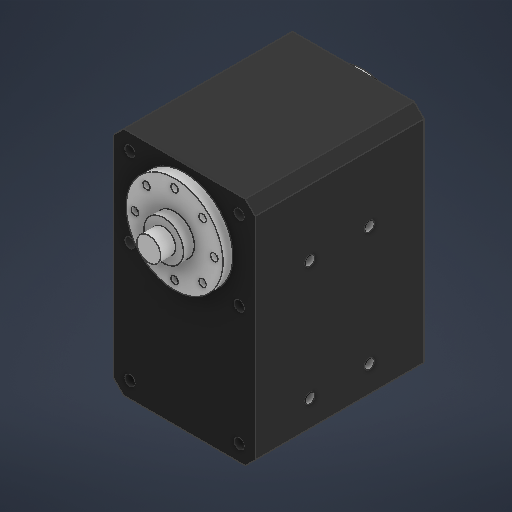
# Autodesk Inventor part: DYNAMIXEL XM430-W350
Saved by Autodesk Inventor 2025 (Build 290162010, 162A)
## iProperties
Created: 2024-06-21
Part Number: DYNAMIXEL XM430-W350
Material: Типовые
Document SubType Name: Modeling
Designer: Edward_Higgins
Density: 1 g/cm^3
Appearance: По умолчанию
Author: Edward_Higgins
Autodesk Inventor part; units mm, degrees
ref_plane "YZ Plane" through (0, 0, 0) normal (1, 0, 0) x (0, 1, 0)
ref_plane "XZ Plane" through (0, 0, 0) normal (0, 1, 0) x (-1, 0, 0)
ref_plane "XY Plane" through (0, 0, 0) normal (0, 0, 1) x (1, 0, 0)
sketch "Эскиз1" plane through (0, 0, 0) normal (0, 0, 1) x (1, 0, 0)
  line L0 (-12.25, 11.25) -> (12.25, 11.25)
  line L1 (14.25, 9.25) -> (14.25, -33.25)
  line L2 (12.25, -35.25) -> (-12.25, -35.25)
  line L3 (-14.25, -33.25) -> (-14.25, 9.25)
  circle A0 centre (-11, 8) radius 1
  circle A1 centre (-11, -8) radius 1
  circle A2 centre (11, 8) radius 1
  circle A3 centre (11, -8) radius 1
  circle A4 centre (11, -32) radius 1
  circle A5 centre (-11, -32) radius 1
  line L4 (-12.25, 11.25) -> (-14.25, 9.25)
  line L5 (12.25, 11.25) -> (14.25, 9.25)
  line L6 (14.25, -33.25) -> (12.25, -35.25)
  line L7 (-12.25, -35.25) -> (-14.25, -33.25)
  point P0 (0, 0)
  point P1 (-14.25, 11.25)
  point P2 (14.25, -35.25)
  point P3 (14.25, 11.25)
  point P4 (-14.25, -35.25)
  point P5 (0, 11.25)
  dimension "d0" = 28.5
  dimension "d1" = 46.5
  dimension "d2" = 11.25
  dimension "d3" = 22
  dimension "d4" = 11
  dimension "d5" = 8
  dimension "d6" = 8
  dimension "d7" = 40
  dimension "d8" = 2
  dimension "d11" = 2
  dimension "d12" = 2
  dimension "d13" = 2
  dimension "d14" = 2
  dimension "d15" = 2
  dimension "d16" = 2
  dimension "d17" = 2
  dimension "d18" = 2
  constraints: 16 end point, 8 point on line, 6 centre point, 5 equal radius, 5 vertical alignment, 3 horizontal alignment, 2 parallel, 1 horizontal, 1 midpoint, 1 perpendicular
  measures "d0" distance between parallel lines of L1 L3
  measures "d1" distance between parallel lines of L2 L0
  measures "d2" distance from line of point (0, 0) L0
  measures "d3" distance of A2.centre A0.centre
  measures "d4" horizontal distance of point (0, 11.25) A2.centre
  measures "d5" vertical distance of point (0, 0) A0.centre
  measures "d6" vertical distance of A1.centre point (0, 0)
  measures "d7" distance of A2.centre A4.centre
  measures "d8" diameter of A5
  measures "d11" distance of L0.start point (-14.25, 11.25)
  measures "d12" distance of L3.end point (-14.25, 11.25)
  measures "d13" distance of L0.end point (14.25, 11.25)
  measures "d14" distance of L1.start point (14.25, 11.25)
  measures "d15" distance of L1.end point (14.25, -35.25)
  measures "d16" distance of L2.start point (14.25, -35.25)
  measures "d17" distance of L2.end point (-14.25, -35.25)
  measures "d18" distance of L3.start point (-14.25, -35.25)
extrude "Выдавливание1" add sketch "Эскиз1" against normal blind 34
sketch "Эскиз2" plane through (0, 0, 0) normal (1, 0, 0) x (0, 1, 0)
  line L0 (0, 0) -> (0, 7.2)
  line L1 (0, 7.2) -> (2.4047, 7.2)
  line L2 (2.4047, 7.2) -> (2.4047, 4.2)
  line L3 (2.4047, 4.2) -> (4, 4.2)
  line L4 (4, 4.2) -> (4, 2)
  line L5 (4, 2) -> (9.75, 2)
  line L6 (9.75, 2) -> (9.75, 0)
  line L7 (9.75, 0) -> (0, 0)
  line L8 (-33.25, -34) -> (9.25, -34) projected
  line L9 (0, -34) -> (9.75, -34)
  line L10 (9.75, -34) -> (9.75, -36)
  line L11 (9.75, -36) -> (0, -36)
  line L12 (0, -36) -> (0, -34)
  point P0 (1.2024, 7.2)
  dimension "d19" = 19.5
  dimension "d20" = 8
  dimension "d21" = 2
  dimension "d22" = 2.2
  dimension "d23" = 2
  dimension "d24" = 19.5
  dimension "d25" = 41.2
  constraints: 24 end point, 7 perpendicular, 2 horizontal, 2 parallel, 2 point on line, 1 midpoint, 1 vertical
  measures "d19" diameter of L6 L0
  measures "d20" diameter of L4 L0
  measures "d21" distance between parallel lines of L7 L5
  measures "d22" distance between parallel lines of L3 L5
  measures "d23" distance between parallel lines of L11 L8
  measures "d24" diameter of L10 L0
  measures "d25" distance from line of point (1.202, 7.2) L9
revolve "Вращение1" add sketch "Эскиз2" angle 360 about axis through (0, 0, 0) along (0, 0, 1)
sketch "Эскиз3" plane through (14.25, -33.25, 0) normal (1, 0, 0) x (0, 0, -1)
  circle A0 centre (11, 29.25) radius 1
  circle A1 centre (11, 5.25) radius 1
  circle A2 centre (23, 29.25) radius 1
  circle A3 centre (23, 5.25) radius 1
  line L0 (0, 0) -> (0, 42.5) projected
  line L1 (-7.2, 35.6547) -> (-7.2, 30.8453) projected
  line L2 (-7.2, 33.25) -> (42.1725, 33.25)
  point P0 (0, 33.25)
  dimension "d27" = 11
  dimension "d28" = 12
  dimension "d29" = 24
  dimension "d30" = 4
  dimension "d31" = 2
  constraints: 4 centre point, 3 equal radius, 2 end point, 2 horizontal alignment, 2 vertical alignment, 1 horizontal, 1 midpoint
  measures "d27" distance from line of L0 A1.centre
  measures "d28" distance of A3.centre A1.centre
  measures "d29" distance of A2.centre A3.centre
  measures "d30" distance from line of L2 A2.centre
  measures "d31" diameter of A2
extrude "Выдавливание2" cut sketch "Эскиз3" against normal up to surface (28.5 mm away)
sketch "Эскиз4" plane through (0, 0, 2) normal (0, 0, 1) x (1, 0, 0)
  circle A0 centre (0, -8) radius 0.75
  point P0 (0, 0)
  dimension "d34" = 1.5
  dimension "d35" = 8
  constraints: 1 centre point, 1 vertical alignment
  measures "d34" diameter of A0
  measures "d35" distance of point (0, 0) A0.centre
extrude "Выдавливание3" cut sketch "Эскиз4" against normal blind 2
pattern_circular "Круговой массив1" count 8 over 360 about axis through (0, 0, 1) along (0, 0, 1) of "Выдавливание3"
equation "\"d4\" = 0.5 * d3"
equation "\"d12\" = d11"
equation "\"d13\" = d11"
equation "\"d14\" = d13"
equation "\"d15\" = d11"
equation "\"d16\" = d15"
equation "\"d17\" = d11"
equation "\"d18\" = d17"
